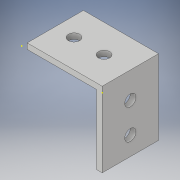
# Autodesk Inventor part: 二つ分け角柱
Saved by Autodesk Inventor 2019 (Build 230136000, 136)
## iProperties
Created: 2020-10-27
Part Number: 二つ分け角柱
Material: 一般
Document SubType Name: Modeling
Designer: X1 Carbon
Density: 1 g/cm^3
Appearance: 既定
Author: X1 Carbon
Autodesk Inventor part; units mm, degrees
ref_plane "YZ Plane" through (0, 0, 0) normal (1, 0, 0) x (0, 1, 0)
ref_plane "XZ Plane" through (0, 0, 0) normal (0, 1, 0) x (-1, 0, 0)
ref_plane "XY Plane" through (0, 0, 0) normal (0, 0, 1) x (1, 0, 0)
sketch "スケッチ1" plane through (0, 0, 0) normal (0, 1, 0) x (-1, 0, 0)
  line L0 (0, 0) -> (20, 0)
  line L1 (20, 0) -> (20, -15)
  line L2 (20, -15) -> (0, -15)
  line L3 (0, -15) -> (0, 0)
  dimension "d0" = 20
  dimension "d1" = 15
  constraints: 8 end point, 2 parallel, 1 horizontal, 1 perpendicular
  measures "d0" distance of L1.end L2.end
  measures "d1" distance of L0.end L1.end
sketch "スケッチ2" plane through (0, 0, 0) normal (1, 0, 0) x (0, 1, 0)
  line L0 (0, 0) -> (-20, 0)
  line L1 (-20, 0) -> (-20, -15)
  line L2 (-20, -15) -> (0, -15)
  line L3 (0, -15) -> (0, 0)
  dimension "d2" = 20
  dimension "d3" = 15
  constraints: 8 end point, 2 parallel, 1 horizontal, 1 perpendicular
  measures "d2" distance of L2.end L1.end
  measures "d3" distance of L1.end L0.end
extrude "押し出し1" add sketch "スケッチ1" along normal blind 1.5
extrude "押し出し2" add sketch "スケッチ2" along normal blind 1.5
sketch "スケッチ3" plane through (0, 0, 0) normal (0, 1, 0) x (1, 0, 0)
  line L0 (0, 15) -> (1.5, 15) projected
  line L1 (0, 0) -> (0, 15) projected
  line L2 (1.5, 15) -> (0, 15)
  line L3 (0, 15) -> (0, 0)
  line L4 (0, 0) -> (1.5, 0)
  line L5 (1.5, 0) -> (1.5, 15)
  constraints: 8 end point, 2 parallel, 1 horizontal, 1 perpendicular
extrude "押し出し3" add sketch "スケッチ3" along normal blind 1.5
sketch "スケッチ4" plane through (1.5, 0, 0) normal (1, 0, 0) x (0, 0, -1)
  point P0 (0, 0)
sketch "スケッチ5" plane through (1.5, 0, 0) normal (1, 0, 0) x (0, 0, -1)
  point P0 (0, 0)
sketch "スケッチ6" plane through (-20, 0, -15) normal (-1, 0, 0) x (0, 0, 1)
  point P0 (15, 0)
sketch "スケッチ7" plane through (-20, 0, -15) normal (-1, 0, 0) x (0, 0, 1)
  line L0 (15.9074, 4.1741) -> (-1.7689, 4.1741)
  line L1 (-1.7689, 4.1741) -> (-1.7689, -3.4482)
  line L2 (-1.7689, -3.4482) -> (15.9074, -3.4482)
  line L3 (15.9074, -3.4482) -> (15.9074, 4.1741)
  point P0 (15, 0)
  constraints: 8 end point, 2 parallel, 1 horizontal, 1 perpendicular
extrude "押し出し4" cut sketch "スケッチ7" against normal blind 1.5
sketch "スケッチ8" plane through (0, -20, -15) normal (0, -1, 0) x (1, 0, 0)
  line L0 (-2.0326, 16.6333) -> (6.4245, 16.6333)
  line L1 (6.4245, 16.6333) -> (6.4245, -1.5875)
  line L2 (6.4245, -1.5875) -> (-2.0326, -1.5875)
  line L3 (-2.0326, -1.5875) -> (-2.0326, 16.6333)
  point P0 (0, 15)
  constraints: 8 end point, 2 parallel, 1 horizontal, 1 perpendicular
extrude "押し出し5" cut sketch "スケッチ8" against normal blind 1.5
sketch "スケッチ9" plane through (0, 1.5, 0) normal (0, 1, 0) x (1, 0, 0)
  circle A0 centre (-13.5, 7.5) radius 1.5
  circle A1 centre (-5.5, 7.5) radius 1.5
  point P0 (0, 0)
  dimension "d14" = 3
  dimension "d15" = 3
  constraints: 2 centre point
  measures "d14" diameter of A0
  measures "d15" diameter of A1
sketch "スケッチ10" plane through (1.5, 0, 0) normal (1, 0, 0) x (0, 0, -1)
  circle A0 centre (7.5, -5.5) radius 1.5
  circle A1 centre (7.5, -13.5) radius 1.5
  point P0 (0, 0)
  dimension "d16" = 3
  dimension "d18" = 3
  constraints: 2 centre point
  measures "d16" diameter of A0
  measures "d18" diameter of A1
extrude "押し出し6" cut sketch "スケッチ10" against normal blind 1.5
extrude "押し出し7" cut sketch "スケッチ9" against normal blind 1.5
